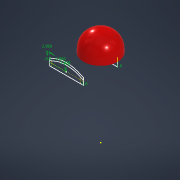
# Autodesk Inventor part: X02598_LEGOmini_Hat_R_Original_NoPara
Saved by Autodesk Inventor 2022 (Build 260153000, 153)
## iProperties
Created: 2015-06-18
Part Number: X02598_LEGOmini_Hat_R_Original_NoPara
Material: ABS Plastic
Document SubType Name: Modeling
Designer: D. Kohfeld
Density: 1.06 g/cm^3
Appearance: Red
Mass: 0.328505 g
Surface Area: 6.75971 cm^2
Volume: 0.309911 cm^3
Author: D. Kohfeld
Autodesk Inventor part; units mm, degrees
ref_plane "YZ Plane" through (0, 0, 0) normal (1, 0, 0) x (0, 1, 0)
ref_plane "XZ Plane" through (0, 0, 0) normal (0, 1, 0) x (-1, 0, 0)
sketch "Sketch2" plane through (0, 0, 0) normal (0, 0, 1) x (1, 0, 0)
  line L0 (0, 6.83) -> (0, 5.9635)
  line L1 (0, 4.4) -> (-2.5, 4.4)
  line L2 (-2.5, 4.4) -> (-2.5, 2.8)
  line L3 (-2.5, 2.8) -> (-3.2, 2.8)
  line L4 (-3.2, 2.8) -> (-3.2, 4.4)
  line L5 (-3.2, 4.4) -> (-3.8296, 4.4)
  line L6 (-6.0665, 0) -> (-5.2, 0)
  line L7 (-5.9942, 1.5241) -> (-6.0665, 0)
  line L8 (-5.1297, 1.4833) -> (-5.2, 0)
  ellipse E0 centre (0, 1.281) end of major axis (0, 6.83) minor radius 6 (0, 6.83) -> (-5.9942, 1.5241) ccw
  ellipse E1 centre (0, 1.281) end of major axis (0, 5.9635) minor radius 5.1345 (-3.8296, 4.4) -> (-5.1297, 1.4833) ccw
  line L9 (0, 5.9635) -> (0, 4.4)
  line L10 (-5.2, 0) -> (0, 0)
  line L11 (0, 0) -> (0, 4.4)
  line L12 (-6.0067, 1.261) -> (6.0067, 1.261) construction
  line L13 (6.0067, 1.261) -> (6.0665, 0) construction
  line L14 (-6.0067, 1.261) -> (-6.0665, 0)
  arc A0 (5.2, 0) -> (-5.2, 0) centre (0, -27.986) ccw construction
  line L15 (5.2, 0) -> (6.0665, 0) construction
  point P0 (0, 1.261)
  dimension "d10" = 6
  dimension "d11" = 5.549
  dimension "d0" = 6.83
  dimension "d1" = 10.4
  dimension "d2" = 12.133
  dimension "d3" = 1.6
  dimension "d4" = 6.4
  dimension "d5" = 5
  dimension "d6" = 4.4
  dimension "d15" = 1.261
  dimension "d18" = 0.479
  constraints: 32 end point, 7 horizontal, 5 vertical, 3 equal length, 3 horizontal alignment, 2 point on circle, 2 point on line, 2 vertical alignment, 1 centre point, 1 coincident, 1 midpoint, 1 parallel, 11 other
  measures "d0" distance of L0.start L10.end
  measures "d1" diameter of L6.end L0
  measures "d2" diameter of L6.start L0
  measures "d3" distance between parallel lines of L1 L3
  measures "d4" diameter of L4 L0
  measures "d5" diameter of L2 L0
  measures "d6" distance from line of L1 L10.end
  measures "d15" distance between parallel lines of L6 L12
  measures "d18" distance edge to line of A0 L10
revolve "Revolution1" add sketch "Sketch2" angle 360 about axis through (0, 6.83, 0) along (0, -1, 0)
ref_plane "Work Plane2" through (0, 0, 12.21) normal (0, 0, 1) x (1, 0, 0)
sketch "Sketch7" plane through (0, 0, 0) normal (0, 0, 1) x (1, 0, 0)
  line L0 (-6.0067, 1.261) -> (-6.0665, 0) projected
  line L1 (-6.0665, 0) -> (-5.2, 0) projected
  arc A0 (5.2, 0) -> (-5.2, 0) centre (0, -27.986) ccw projected
  line L2 (5.2, 0) -> (6.0665, 0) projected
  line L3 (6.0067, 1.261) -> (6.0665, 0) projected
  line L4 (-6.0067, 1.261) -> (6.0067, 1.261) projected
  line L5 (-6.0665, 0) -> (-6.0665, -1.6)
  line L6 (-6.0665, -1.6) -> (6.0665, -1.6)
  line L7 (6.0665, -1.6) -> (6.0665, 0)
  point P0 (0, 0)
  dimension "d42" = 1.6
  constraints: 6 end point, 2 vertical, 1 horizontal
  measures "d42" distance between parallel lines of L6 L2
sketch "Sketch6" plane through (0, 0, 12.21) normal (0, 0, 1) x (1, 0, 0)
  line L0 (-6.0067, 1.261) -> (-6.0665, 0) construction
  line L1 (6.0067, 1.261) -> (6.0665, 0) construction
  line L2 (-6.0665, 1.2363) -> (-6.0665, 0.4363)
  line L3 (6.0665, 1.2363) -> (6.0665, 0.4363)
  line L4 (6.0665, 0) -> (-6.0665, 0) construction
  line L5 (-6.0665, 1.2363) -> (-3.9179, 2.123)
  line L6 (6.0665, 1.2363) -> (3.9179, 2.123)
  line L7 (-6.0665, 0.4363) -> (-3.7812, 1.3794)
  line L8 (6.0665, 0.4363) -> (3.7812, 1.3794)
  ellipse E0 centre (0, -0.136) end of major axis (5.3087, -0.136) minor radius 2.159 (3.7812, 1.3794) -> (-3.7812, 1.3794) ccw
  ellipse E1 centre (0, -0.136) end of major axis (0, 2.823) minor radius 6.066 (3.9179, 2.123) -> (-3.9179, 2.123) ccw
  line L9 (0, 2.823) -> (0, 2.023) construction
  line L10 (-6.0665, 0.4363) -> (-6.0665, -1.1637)
  line L11 (-6.0665, -1.1637) -> (6.0665, -1.1637)
  line L12 (6.0665, -1.1637) -> (6.0665, 0.4363)
  point P0 (0, 0)
  point P1 (-5.2, 0)
  point P2 (5.2, 0)
  point P3 (0, 0)
  dimension "d33" = 6.066
  dimension "d34" = 2.959
  dimension "d31" = 0.8
  dimension "d32" = 2.823
  dimension "d35" = 0.8
  dimension "d41" = 1.6
  constraints: 20 end point, 5 vertical, 4 point on line, 2 horizontal alignment, 2 parallel, 1 coincident, 1 equal length, 1 horizontal, 1 midpoint, 1 vertical alignment, 14 other
  measures "d31" distance of L9.start L9.end
  measures "d32" distance from line of L9.start L4
  measures "d35" distance of L2.start L2.end
  measures "d41" distance from line of L3.end L11
revolve "Revolution2" cut sketch "Sketch2" angle 360 about axis through (0, 0, 0) along (0, 1, 0) contours L11 L10 L8 E1 L5 L4 L3 L2 L1
sketch "Sketch4" plane through (0, 2.8, 0) normal (0, -1, 0) x (1, 0, 0)
  line L0 (-3.1432, 0.6) -> (-2.4269, 0.6)
  line L1 (2.4269, 0.6) -> (3.1432, 0.6)
  line L2 (-3.1432, -0.6) -> (-2.4269, -0.6)
  line L3 (2.4269, -0.6) -> (3.1432, -0.6)
  circle A0 centre (0, 0) radius 3.2 projected
  circle A1 centre (0, 0) radius 2.5 projected
  dimension "d12" = 1.2
  constraints: 8 end point, 8 point on circle, 4 horizontal, 3 equal length
  measures "d12" distance between parallel lines of L2 L0
extrude "Extrusion1" cut sketch "Sketch4" against normal up to surface (1.6 mm away) contours L0 A1 L2 A0 | A0 L3 A1 L1
sketch "Sketch8" plane through (0, 0, 0) normal (1, 0, 0) x (0, 1, 0)
  line L0 (0, -6.0665) -> (0, 0) projected
  line L1 (0, -6.0665) -> (1.5241, -5.9942) construction
  line L2 (0, 0) -> (0.121, -6.0608)
  line L3 (0.121, -6.0608) -> (0, -6.0665)
  dimension "d47" = 0.121
  constraints: 4 end point, 1 collinear, 1 point on line
  measures "d47" distance from line of L2.end L0
extrude "Extrusion2" cut sketch "Sketch8" along normal through all both and the other way through all
sketch "草圖10" plane through (0, 0, 0) normal (0, 0, 1) x (1, 0, 0)
  ellipse E0 centre (0, -0.0001) end of major axis (-6.0665, -0.0001) minor radius 0.1211 (6.0665, 0) -> (-6.0665, 0) ccw projected
  point P0 (0, 0)
  constraints: 1 other
sketch "草圖11" plane through (0, 0, 0) normal (0, 0, 1) x (1, 0, 0)
  ellipse E0 centre (0, 1.281) end of major axis (-6, 1.281) minor radius 5.549 (0, 6.83) -> (-5.9942, 1.5241) ccw construction
  line L0 (5.9942, 1.5241) -> (-5.9942, 1.5241) construction
  ellipse E1 centre (0, -0.0001) end of major axis (-5.2, -0.0001) minor radius 0.1038 (5.2, 0) -> (-5.2, 0) ccw construction
  line L1 (0, -0.0001) -> (0, 6.83) construction
  circle A0 centre (-10.4351, 2.8) radius 1.75
  line L2 (-2.4269, 2.8) -> (2.4269, 2.8) projected
  point P0 (0, 0)
  point P1 (0, 2.8)
  dimension "d54" = 6.8301
  dimension "d55" = 3.5
  constraints: 2 end point, 1 centre point, 1 horizontal alignment, 1 midpoint, 1 vertical, 2 other
  measures "d54" distance of L1.start L1.end
  measures "d55" diameter of A0
revolve "迴轉3" add sketch "草圖11" angle 360 about axis through (0, -0.0001, 0) along (0, 1, 0)
equation "\"topthk\" = 1.6"
body "Solid1"
